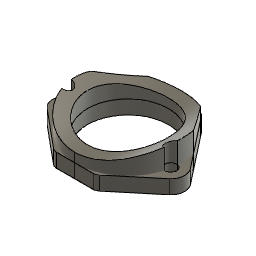
110mm Dia MAF Mount v4 (Autodesk Fusion 360 design; units mm, degrees)
Autodesk Fusion 360 part; units mm, degrees
note: some values were not read from the file. Chosen so that the rebuilt part matches the saved one: which face or edge a step refers to; which pieces of a blend or face edit are solid. Set by a fixed rule: which sketch regions a step uses.
sketch "Sketch1" plane through (0, 0, 0) normal (0, 1, 0) x (1, 0, 0)
  circle A0 centre (0, 0) radius 17.5
  circle A1 centre (0, 0) radius 23
  line L0 (0, -10) -> (0, -11)
  circle A2 centre (22.5, -4) radius 2.5
  circle A3 centre (-22.5, -4) radius 2.5
  line L1 (0.0078, -23) -> (-8.9922, -23)
  line L2 (0.0078, -23) -> (9.0078, -23)
  line L3 (-0.009, 23) -> (-9.009, 22.9931)
  line L4 (-0.009, 23) -> (8.991, 23.0069)
  circle A4 centre (-22.5, -4) radius 6
  circle A5 centre (22.5, -4) radius 6
  line L5 (-9.009, 22.9931) -> (-27.2265, -0.304)
  line L6 (8.991, 23.0069) -> (27.2258, -0.3031)
  line L7 (9.0078, -23) -> (26.3327, -8.6164)
  line L8 (-8.9922, -23) -> (-26.3306, -8.6181)
  dimension "d1" = 35
  dimension "d2" = 46
  dimension "d6" = 5
  dimension "d7" = 5
  dimension "d8" = 9
  dimension "d9" = 9
  dimension "d10" = 9
  dimension "d11" = 9
  dimension "d12" = 12
  dimension "d13" = 12
  constraint coincident A0.centre A1.centre
  constraint concentric A0 A1
  constraint coincident A1 L1.start
  constraint horizontal L1
  constraint parallel L1 L2
  constraint coincident A1 L3.start
  constraint parallel L3 L4
  constraint concentric A3 A4
  constraint concentric A2 A5
  constraint coincident A4 L5.end
  constraint tangent A4 L5
  constraint coincident A5 L6.end
  constraint tangent A5 L6
  constraint coincident A5 L7.end
  constraint tangent A5 L7
  constraint coincident A4 L8.end
  constraint tangent A4 L8
  measures "d1" diameter of A0
  measures "d2" diameter of A1
  measures "d6" diameter of A2
  measures "d7" diameter of A3
  measures "d8" distance of L1.start L1.end
  measures "d9" distance of L1.start L2.end
  measures "d10" distance of L3.start L3.end
  measures "d11" distance of L3.start L4.end
  measures "d12" diameter of A4
  measures "d13" diameter of A5
sketch "Sketch2" plane through (0, 0, 0) normal (0, 0, 1) x (1, 0, 0)
  circle A0 centre (0, 64.96) radius 55
  dimension "d18" = 110
  measures "d18" diameter of A0
extrude "Extrude11" add sketch "Sketch1" along normal blind 28 contours A0 A1 A4 A5 L5 L6 makes body 1
extrude "Extrude13" cut sketch "Sketch2" against normal blind 66 bodies 1
extrude "Extrude14" cut sketch "Sketch2" along normal blind 25 bodies 1
fillet "Fillet8" radius 3 1 edges at (22.9141, 7.4803, -1.9857) on bodies 1
fillet "Fillet10" radius 3 3 edges at (-22.6321, 14.8323, -4.0973) (-22.9141, 7.4803, -1.9857) (-22.6311, 0, -4.1026) on bodies 1
delete_body "RemoveBody1" bodies 1
extrude "Extrude15" add sketch "Sketch1" along normal blind 6 separate body contours A1 L3 L5 | A0 A1 A4 A5 L5 L6 | A0 A1 A3 A4 | A0 A1 A2 A5 | A0 A1 A4 A5 | A1 A4 L5 | A1 A3 A4 | A1 A2 A5 | A1 A5 L6 | A1 L2 A5 L7 | A1 L1 A4 L8 | A1 L4 L6 makes body 2
extrude "Extrude16" add sketch "Sketch1" along normal blind 28 separate body contours A0 A1 A4 A5 L5 L6 | A0 A1 A3 A4 | A0 A1 A2 A5 | A0 A1 A4 A5 makes body 3
extrude "Extrude17" cut sketch "Sketch2" along normal blind 140 bodies 3
extrude "Extrude18" cut sketch "Sketch2" against normal blind 37 bodies 3
fillet "Fillet12" radius 3 4 edges at (-8.9922, 3, 23) (9.0078, 3, 23) (8.991, 3, -23.0069) (-9.009, 3, -22.9931) on bodies 2
